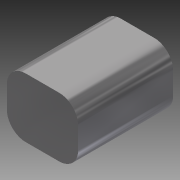
# Autodesk Inventor part: Gearmotor_Motor
Saved by Autodesk Inventor 2013 (Build 170138000, 138)
## iProperties
Created: 2015-07-02
Part Number: Gearmotor_Motor
Material: Stainless Steel
Document SubType Name: Modeling
Designer: Kyle
Density: 8.08 g/cm^3
Mass: 1.65716 g
Surface Area: 16.1532 cm^2
Volume: 0.205094 cm^3
Author: Kyle
Autodesk Inventor part; units mm, degrees
ref_plane "YZ Plane" through (0, 0, 0) normal (1, 0, 0) x (0, 1, 0)
ref_plane "XZ Plane" through (0, 0, 0) normal (0, 1, 0) x (-1, 0, 0)
ref_plane "XY Plane" through (0, 0, 0) normal (0, 0, 1) x (1, 0, 0)
sketch "Sketch1" plane through (0, 0, 0) normal (0, 0, 1) x (1, 0, 0)
  line L0 (0, 0) -> (11.9888, 0)
  line L1 (11.9888, 0) -> (11.9888, 10.0076)
  line L2 (11.9888, 10.0076) -> (0, 10.0076)
  line L3 (0, 10.0076) -> (0, 0)
  dimension "d0" = 10.0076
  dimension "d1" = 11.9888
  constraints: 8 end point, 2 parallel, 1 horizontal, 1 perpendicular
  measures "d0" distance of L2.end L0.start
  measures "d1" distance of L1.end L2.end
extrude "Extrusion1" add sketch "Sketch1" along normal blind 16.002
fillet "Fillet1" radius 3.175 4 edges at (11.9888, 10.0076, 8.001) (0, 10.0076, 8.001) (11.9888, 0, 8.001) (0, 0, 8.001)
shell "Shell2" thickness 0.254 removed faces 0
body "Solid1"
